Autodesk Fusion 360 part; units mm, degrees
(part 23 of 25)
sketch "Bottom Component Outlines" plane through (0, 0, 0) normal (0, 0, 1) x (1, 0, 0)
  arc A0 (46.3191, 48.2959) -> (46.3909, 48.2241) centre (46.355, 48.26) ccw
  line L0 (59.055, 7.62) -> (57.785, 7.62)
  arc A1 (67.9809, 7.5841) -> (67.9091, 7.6559) centre (67.945, 7.62) ccw
  arc A2 (67.2741, 7.0209) -> (67.3459, 6.9491) centre (67.31, 6.985) ccw
  arc A3 (52.705, 7.6708) -> (52.705, 7.5692) centre (52.705, 7.62) ccw
  arc A4 (53.9391, 5.1159) -> (54.0109, 5.0441) centre (53.975, 5.08) ccw
  arc A5 (51.3991, 5.1159) -> (51.4709, 5.0441) centre (51.435, 5.08) ccw
  arc A6 (49.4941, 7.0209) -> (49.5659, 6.9491) centre (49.53, 6.985) ccw
  arc A7 (69.215, 7.5692) -> (69.215, 7.6708) centre (69.215, 7.62) ccw
  arc A8 (49.5659, 5.7509) -> (49.4941, 5.6791) centre (49.53, 5.715) ccw
  arc A9 (52.705, 5.1308) -> (52.705, 5.0292) centre (52.705, 5.08) ccw
  arc A10 (67.9091, 5.0441) -> (67.9809, 5.1159) centre (67.945, 5.08) ccw
  arc A11 (54.5741, 6.9491) -> (54.6459, 7.0209) centre (54.61, 6.985) ccw
  line L1 (52.07, 6.985) -> (51.435, 7.62)
  line L2 (54.61, 6.985) -> (53.975, 7.62)
  line L3 (52.07, 5.715) -> (52.705, 5.08)
  line L4 (51.435, 5.08) -> (52.07, 5.715)
  arc A12 (52.7409, 7.5841) -> (52.6691, 7.6559) centre (52.705, 7.62) ccw
  arc A13 (50.1291, 5.0441) -> (50.2009, 5.1159) centre (50.165, 5.08) ccw
  arc A14 (54.6459, 5.6791) -> (54.5741, 5.7509) centre (54.61, 5.715) ccw
  arc A15 (69.7992, 5.715) -> (69.9008, 5.715) centre (69.85, 5.715) ccw
  arc A16 (51.4709, 7.6559) -> (51.3991, 7.5841) centre (51.435, 7.62) ccw
  arc A17 (46.3909, 50.8359) -> (46.3191, 50.7641) centre (46.355, 50.8) ccw
  line L5 (69.85, 6.985) -> (69.215, 7.62)
  arc A18 (52.1059, 5.7509) -> (52.0341, 5.6791) centre (52.07, 5.715) ccw
  line L6 (69.85, 5.715) -> (69.85, 6.985)
  arc A19 (69.1791, 5.1159) -> (69.2509, 5.0441) centre (69.215, 5.08) ccw
  arc A20 (54.0109, 7.6559) -> (53.9391, 7.5841) centre (53.975, 7.62) ccw
  line L7 (52.705, 5.08) -> (53.975, 5.08)
  arc A21 (52.0341, 7.0209) -> (52.1059, 6.9491) centre (52.07, 6.985) ccw
  arc A22 (69.2509, 7.6559) -> (69.1791, 7.5841) centre (69.215, 7.62) ccw
  line L8 (45.085, 48.26) -> (46.355, 48.26)
  arc A23 (52.705, 50.8508) -> (52.705, 50.7492) centre (52.705, 50.8) ccw
  arc A24 (69.9008, 6.985) -> (69.7992, 6.985) centre (69.85, 6.985) ccw
  line L9 (67.31, 6.985) -> (67.945, 7.62)
  arc A25 (53.975, 7.5692) -> (53.975, 7.6708) centre (53.975, 7.62) ccw
  line L10 (52.705, 7.62) -> (52.07, 6.985)
  arc A26 (52.1059, 5.6791) -> (52.0341, 5.7509) centre (52.07, 5.715) ccw
  arc A27 (52.6691, 5.0441) -> (52.7409, 5.1159) centre (52.705, 5.08) ccw
  line L11 (53.975, 7.62) -> (52.705, 7.62)
  arc A28 (51.435, 7.5692) -> (51.435, 7.6708) centre (51.435, 7.62) ccw
  arc A29 (67.945, 5.1308) -> (67.945, 5.0292) centre (67.945, 5.08) ccw
  line L12 (69.215, 5.08) -> (69.85, 5.715)
  arc A30 (50.165, 5.1308) -> (50.165, 5.0292) centre (50.165, 5.08) ccw
  arc A31 (57.785, 7.6708) -> (57.785, 7.5692) centre (57.785, 7.62) ccw
  arc A32 (47.0259, 48.8591) -> (46.9541, 48.9309) centre (46.99, 48.895) ccw
  arc A33 (59.055, 7.5692) -> (59.055, 7.6708) centre (59.055, 7.62) ccw
  arc A34 (69.215, 5.0292) -> (69.215, 5.1308) centre (69.215, 5.08) ccw
  arc A35 (51.435, 5.0292) -> (51.435, 5.1308) centre (51.435, 5.08) ccw
  line L13 (53.975, 5.08) -> (54.61, 5.715)
  line L14 (51.435, 7.62) -> (50.165, 7.62)
  line L15 (50.165, 5.08) -> (49.53, 5.715)
  line L16 (69.215, 7.62) -> (67.945, 7.62)
  arc A36 (67.945, 7.6708) -> (67.945, 7.5692) centre (67.945, 7.62) ccw
  line L17 (67.945, 5.08) -> (67.31, 5.715)
  arc A37 (50.2009, 7.5841) -> (50.1291, 7.6559) centre (50.165, 7.62) ccw
  arc A38 (50.165, 7.6708) -> (50.165, 7.5692) centre (50.165, 7.62) ccw
  line L18 (52.07, 48.895) -> (52.705, 48.26)
  arc A39 (52.0341, 6.9491) -> (52.1059, 7.0209) centre (52.07, 6.985) ccw
  line L19 (67.945, 5.08) -> (69.215, 5.08)
  line L20 (50.165, 5.08) -> (51.435, 5.08)
  line L21 (49.53, 6.985) -> (50.165, 7.62)
  arc A40 (67.3459, 5.7509) -> (67.2741, 5.6791) centre (67.31, 5.715) ccw
  arc A41 (69.8859, 5.6791) -> (69.8141, 5.7509) centre (69.85, 5.715) ccw
  arc A42 (52.0341, 50.2009) -> (52.1059, 50.1291) centre (52.07, 50.165) ccw
  arc A43 (46.9541, 50.2009) -> (47.0259, 50.1291) centre (46.99, 50.165) ccw
  line L22 (53.975, 50.8) -> (52.705, 50.8)
  arc A44 (46.355, 48.2092) -> (46.355, 48.3108) centre (46.355, 48.26) ccw
  arc A45 (45.0491, 48.2241) -> (45.1209, 48.2959) centre (45.085, 48.26) ccw
  arc A46 (48.895, 50.7492) -> (48.895, 50.8508) centre (48.895, 50.8) ccw
  arc A47 (45.085, 48.3108) -> (45.085, 48.2092) centre (45.085, 48.26) ccw
  line L23 (48.895, 50.8) -> (47.625, 50.8)
  line L24 (46.355, 50.8) -> (45.085, 50.8)
  line L25 (47.625, 50.8) -> (46.99, 50.165)
  arc A48 (49.4941, 50.1291) -> (49.5659, 50.2009) centre (49.53, 50.165) ccw
  line L26 (44.45, 48.895) -> (45.085, 48.26)
  arc A49 (49.5659, 48.8591) -> (49.4941, 48.9309) centre (49.53, 48.895) ccw
  arc A50 (46.9541, 50.1291) -> (47.0259, 50.2009) centre (46.99, 50.165) ccw
  arc A51 (44.4859, 48.9309) -> (44.4141, 48.8591) centre (44.45, 48.895) ccw
  arc A52 (45.1209, 50.7641) -> (45.0491, 50.8359) centre (45.085, 50.8) ccw
  arc A53 (50.2009, 50.7641) -> (50.1291, 50.8359) centre (50.165, 50.8) ccw
  arc A54 (44.4141, 50.2009) -> (44.4859, 50.1291) centre (44.45, 50.165) ccw
  line L27 (49.53, 50.165) -> (48.895, 50.8)
  line L28 (47.625, 48.26) -> (48.895, 48.26)
  line L29 (55.245, 48.26) -> (56.515, 48.26)
  arc A55 (47.0259, 48.9309) -> (46.9541, 48.8591) centre (46.99, 48.895) ccw
  line L30 (52.07, 50.165) -> (51.435, 50.8)
  line L31 (45.085, 50.8) -> (44.45, 50.165)
  arc A56 (52.7409, 50.7641) -> (52.6691, 50.8359) centre (52.705, 50.8) ccw
  arc A57 (47.6609, 50.7641) -> (47.5891, 50.8359) centre (47.625, 50.8) ccw
  arc A58 (46.355, 50.7492) -> (46.355, 50.8508) centre (46.355, 50.8) ccw
  line L32 (49.53, 48.895) -> (50.165, 48.26)
  arc A59 (55.2091, 48.2241) -> (55.2809, 48.2959) centre (55.245, 48.26) ccw
  arc A60 (47.5891, 48.2241) -> (47.6609, 48.2959) centre (47.625, 48.26) ccw
  line L33 (46.99, 48.895) -> (46.355, 48.26)
  line L34 (56.515, 50.8) -> (55.245, 50.8)
  arc A61 (53.975, 48.2092) -> (53.975, 48.3108) centre (53.975, 48.26) ccw
  arc A62 (48.8591, 48.2959) -> (48.9309, 48.2241) centre (48.895, 48.26) ccw
  arc A63 (48.895, 48.2092) -> (48.895, 48.3108) centre (48.895, 48.26) ccw
  line L35 (52.705, 50.8) -> (52.07, 50.165)
  arc A64 (47.625, 50.8508) -> (47.625, 50.7492) centre (47.625, 50.8) ccw
  arc A65 (48.9309, 50.8359) -> (48.8591, 50.7641) centre (48.895, 50.8) ccw
  arc A66 (53.975, 50.7492) -> (53.975, 50.8508) centre (53.975, 50.8) ccw
  arc A67 (45.085, 50.8508) -> (45.085, 50.7492) centre (45.085, 50.8) ccw
  arc A68 (47.625, 48.3108) -> (47.625, 48.2092) centre (47.625, 48.26) ccw
  line L36 (46.99, 48.895) -> (47.625, 48.26)
  line L37 (48.895, 48.26) -> (49.53, 48.895)
  line L38 (46.355, 50.8) -> (46.99, 50.165)
  arc A69 (59.055, 50.7492) -> (59.055, 50.8508) centre (59.055, 50.8) ccw
  arc A70 (51.435, 50.7492) -> (51.435, 50.8508) centre (51.435, 50.8) ccw
  arc A71 (50.165, 50.8508) -> (50.165, 50.7492) centre (50.165, 50.8) ccw
  arc A72 (56.515, 50.7492) -> (56.515, 50.8508) centre (56.515, 50.8) ccw
  line L39 (59.055, 50.8) -> (57.785, 50.8)
  line L40 (50.165, 50.8) -> (49.53, 50.165)
  arc A73 (59.6541, 50.1291) -> (59.7259, 50.2009) centre (59.69, 50.165) ccw
  arc A74 (61.595, 50.7492) -> (61.595, 50.8508) centre (61.595, 50.8) ccw
  arc A75 (52.1059, 48.9309) -> (52.0341, 48.8591) centre (52.07, 48.895) ccw
  line L41 (54.61, 48.895) -> (55.245, 48.26)
  arc A76 (54.6459, 48.8591) -> (54.5741, 48.9309) centre (54.61, 48.895) ccw
  arc A77 (55.245, 50.8508) -> (55.245, 50.7492) centre (55.245, 50.8) ccw
  arc A78 (60.2891, 48.2241) -> (60.3609, 48.2959) centre (60.325, 48.26) ccw
  arc A79 (52.6691, 48.2241) -> (52.7409, 48.2959) centre (52.705, 48.26) ccw
  arc A80 (60.3609, 50.7641) -> (60.2891, 50.8359) centre (60.325, 50.8) ccw
  arc A81 (52.0341, 50.1291) -> (52.1059, 50.2009) centre (52.07, 50.165) ccw
  arc A82 (51.4709, 50.8359) -> (51.3991, 50.7641) centre (51.435, 50.8) ccw
  line L42 (61.595, 50.8) -> (60.325, 50.8)
  line L43 (51.435, 50.8) -> (50.165, 50.8)
  arc A83 (57.1141, 50.1291) -> (57.1859, 50.2009) centre (57.15, 50.165) ccw
  line L44 (57.15, 50.165) -> (56.515, 50.8)
  arc A84 (50.165, 48.3108) -> (50.165, 48.2092) centre (50.165, 48.26) ccw
  arc A85 (55.2809, 50.7641) -> (55.2091, 50.8359) centre (55.245, 50.8) ccw
  line L45 (51.435, 48.26) -> (52.07, 48.895)
  arc A86 (57.1141, 50.2009) -> (57.1859, 50.1291) centre (57.15, 50.165) ccw
  arc A87 (51.435, 48.2092) -> (51.435, 48.3108) centre (51.435, 48.26) ccw
  arc A88 (55.245, 48.3108) -> (55.245, 48.2092) centre (55.245, 48.26) ccw
  arc A89 (52.705, 48.3108) -> (52.705, 48.2092) centre (52.705, 48.26) ccw
  arc A90 (60.325, 50.8508) -> (60.325, 50.7492) centre (60.325, 50.8) ccw
  line L46 (59.69, 48.895) -> (60.325, 48.26)
  arc A91 (49.5659, 48.9309) -> (49.4941, 48.8591) centre (49.53, 48.895) ccw
  line L47 (54.61, 48.895) -> (53.975, 48.26)
  line L48 (50.165, 48.26) -> (51.435, 48.26)
  line L49 (57.785, 50.8) -> (57.15, 50.165)
  arc A92 (56.5509, 50.8359) -> (56.4791, 50.7641) centre (56.515, 50.8) ccw
  arc A93 (54.5741, 50.1291) -> (54.6459, 50.2009) centre (54.61, 50.165) ccw
  arc A94 (49.4941, 50.2009) -> (49.5659, 50.1291) centre (49.53, 50.165) ccw
  arc A95 (53.9391, 48.2959) -> (54.0109, 48.2241) centre (53.975, 48.26) ccw
  arc A96 (52.1059, 48.8591) -> (52.0341, 48.9309) centre (52.07, 48.895) ccw
  line L50 (52.705, 48.26) -> (53.975, 48.26)
  arc A97 (54.6459, 48.9309) -> (54.5741, 48.8591) centre (54.61, 48.895) ccw
  arc A98 (54.5741, 50.2009) -> (54.6459, 50.1291) centre (54.61, 50.165) ccw
  arc A99 (57.785, 50.8508) -> (57.785, 50.7492) centre (57.785, 50.8) ccw
  arc A100 (57.1859, 48.8591) -> (57.1141, 48.9309) centre (57.15, 48.895) ccw
  arc A101 (59.0191, 48.2959) -> (59.0909, 48.2241) centre (59.055, 48.26) ccw
  arc A102 (51.3991, 48.2959) -> (51.4709, 48.2241) centre (51.435, 48.26) ccw
  line L51 (57.785, 48.26) -> (59.055, 48.26)
  line L52 (60.325, 50.8) -> (59.69, 50.165)
  arc A103 (54.0109, 50.8359) -> (53.9391, 50.7641) centre (53.975, 50.8) ccw
  line L53 (56.515, 48.26) -> (57.15, 48.895)
  line L54 (59.69, 50.165) -> (59.055, 50.8)
  arc A104 (59.0909, 50.8359) -> (59.0191, 50.7641) centre (59.055, 50.8) ccw
  line L55 (55.245, 50.8) -> (54.61, 50.165)
  arc A105 (28.575, 50.7492) -> (28.575, 50.8508) centre (28.575, 50.8) ccw
  arc A106 (26.7059, 48.9309) -> (26.6341, 48.8591) centre (26.67, 48.895) ccw
  arc A107 (29.2459, 48.9309) -> (29.1741, 48.8591) centre (29.21, 48.895) ccw
  arc A108 (26.6341, 50.2009) -> (26.7059, 50.1291) centre (26.67, 50.165) ccw
  arc A109 (31.1509, 50.8359) -> (31.0791, 50.7641) centre (31.115, 50.8) ccw
  line L56 (34.925, 50.8) -> (34.29, 50.165)
  arc A110 (56.4791, 48.2959) -> (56.5509, 48.2241) centre (56.515, 48.26) ccw
  line L57 (28.575, 50.8) -> (29.21, 50.165)
  arc A111 (56.515, 48.2092) -> (56.515, 48.3108) centre (56.515, 48.26) ccw
  arc A112 (57.785, 48.3108) -> (57.785, 48.2092) centre (57.785, 48.26) ccw
  arc A113 (62.2659, 48.8591) -> (62.1941, 48.9309) centre (62.23, 48.895) ccw
  line L58 (29.21, 48.895) -> (28.575, 48.26)
  arc A114 (29.1741, 50.2009) -> (29.2459, 50.1291) centre (29.21, 50.165) ccw
  line L59 (59.055, 48.26) -> (59.69, 48.895)
  line L60 (29.845, 48.26) -> (31.115, 48.26)
  arc A115 (50.1291, 48.2241) -> (50.2009, 48.2959) centre (50.165, 48.26) ccw
  arc A116 (62.1941, 50.1291) -> (62.2659, 50.2009) centre (62.23, 50.165) ccw
  arc A117 (62.1792, 48.895) -> (62.2808, 48.895) centre (62.23, 48.895) ccw
  arc A118 (34.9609, 50.7641) -> (34.8891, 50.8359) centre (34.925, 50.8) ccw
  arc A119 (31.115, 48.2092) -> (31.115, 48.3108) centre (31.115, 48.26) ccw
  line L61 (29.845, 50.8) -> (29.21, 50.165)
  line L62 (31.75, 50.165) -> (31.115, 50.8)
  line L63 (27.305, 50.8) -> (26.67, 50.165)
  arc A120 (59.6541, 50.2009) -> (59.7259, 50.1291) centre (59.69, 50.165) ccw
  arc A121 (27.3409, 50.7641) -> (27.2691, 50.8359) centre (27.305, 50.8) ccw
  arc A122 (57.7491, 48.2241) -> (57.8209, 48.2959) centre (57.785, 48.26) ccw
  arc A123 (34.2541, 50.2009) -> (34.3259, 50.1291) centre (34.29, 50.165) ccw
  arc A124 (61.595, 48.2092) -> (61.595, 48.3108) centre (61.595, 48.26) ccw
  arc A125 (31.115, 50.7492) -> (31.115, 50.8508) centre (31.115, 50.8) ccw
  line L64 (53.975, 50.8) -> (54.61, 50.165)
  arc A126 (62.2808, 50.165) -> (62.1792, 50.165) centre (62.23, 50.165) ccw
  arc A127 (59.7259, 48.9309) -> (59.6541, 48.8591) centre (59.69, 48.895) ccw
  arc A128 (34.925, 50.8508) -> (34.925, 50.7492) centre (34.925, 50.8) ccw
  line L65 (62.23, 50.165) -> (62.23, 48.895)
  line L66 (62.23, 48.895) -> (61.595, 48.26)
  arc A129 (59.7259, 48.8591) -> (59.6541, 48.9309) centre (59.69, 48.895) ccw
  arc A130 (36.8659, 48.8591) -> (36.7941, 48.9309) centre (36.83, 48.895) ccw
  arc A131 (37.465, 48.3108) -> (37.465, 48.2092) centre (37.465, 48.26) ccw
  arc A132 (36.8659, 48.9309) -> (36.7941, 48.8591) centre (36.83, 48.895) ccw
  arc A133 (39.4059, 48.8591) -> (39.3341, 48.9309) centre (39.37, 48.895) ccw
  line L67 (57.15, 48.895) -> (57.785, 48.26)
  arc A134 (60.325, 48.3108) -> (60.325, 48.2092) centre (60.325, 48.26) ccw
  arc A135 (29.8809, 50.7641) -> (29.8091, 50.8359) centre (29.845, 50.8) ccw
  arc A136 (29.2459, 48.8591) -> (29.1741, 48.9309) centre (29.21, 48.895) ccw
  line L68 (60.325, 48.26) -> (61.595, 48.26)
  line L69 (29.21, 48.895) -> (29.845, 48.26)
  line L70 (31.115, 48.26) -> (31.75, 48.895)
  arc A137 (29.845, 50.8508) -> (29.845, 50.7492) centre (29.845, 50.8) ccw
  arc A138 (61.5591, 48.2959) -> (61.6309, 48.2241) centre (61.595, 48.26) ccw
  arc A139 (34.3259, 48.8591) -> (34.2541, 48.9309) centre (34.29, 48.895) ccw
  line L71 (34.29, 50.165) -> (33.655, 50.8)
  arc A140 (43.815, 50.7492) -> (43.815, 50.8508) centre (43.815, 50.8) ccw
  arc A141 (57.8209, 50.7641) -> (57.7491, 50.8359) centre (57.785, 50.8) ccw
  line L72 (32.385, 50.8) -> (31.75, 50.165)
  arc A142 (61.6309, 50.8359) -> (61.5591, 50.7641) centre (61.595, 50.8) ccw
  line L73 (27.305, 48.26) -> (28.575, 48.26)
  arc A143 (27.305, 50.8508) -> (27.305, 50.7492) centre (27.305, 50.8) ccw
  line L74 (36.195, 50.8) -> (36.83, 50.165)
  line L75 (31.115, 50.8) -> (29.845, 50.8)
  arc A144 (28.5391, 48.2959) -> (28.6109, 48.2241) centre (28.575, 48.26) ccw
  arc A145 (31.7141, 50.1291) -> (31.7859, 50.2009) centre (31.75, 50.165) ccw
  arc A146 (29.8091, 48.2241) -> (29.8809, 48.2959) centre (29.845, 48.26) ccw
  line L76 (26.67, 48.895) -> (27.305, 48.26)
  arc A147 (57.1859, 48.9309) -> (57.1141, 48.8591) centre (57.15, 48.895) ccw
  arc A148 (31.7859, 48.8591) -> (31.7141, 48.9309) centre (31.75, 48.895) ccw
  arc A149 (34.2541, 50.1291) -> (34.3259, 50.2009) centre (34.29, 50.165) ccw
  line L77 (28.575, 50.8) -> (27.305, 50.8)
  line L78 (36.195, 50.8) -> (34.925, 50.8)
  arc A150 (29.1741, 50.1291) -> (29.2459, 50.2009) centre (29.21, 50.165) ccw
  arc A151 (31.0791, 48.2959) -> (31.1509, 48.2241) centre (31.115, 48.26) ccw
  arc A152 (27.2691, 48.2241) -> (27.3409, 48.2959) centre (27.305, 48.26) ccw
  arc A153 (36.195, 50.7492) -> (36.195, 50.8508) centre (36.195, 50.8) ccw
  line L79 (36.83, 48.895) -> (37.465, 48.26)
  arc A154 (28.6109, 50.8359) -> (28.5391, 50.7641) centre (28.575, 50.8) ccw
  line L80 (33.655, 50.8) -> (32.385, 50.8)
  arc A155 (41.9459, 48.9309) -> (41.8741, 48.8591) centre (41.91, 48.895) ccw
  arc A156 (29.845, 48.3108) -> (29.845, 48.2092) centre (29.845, 48.26) ccw
  arc A157 (59.055, 48.2092) -> (59.055, 48.3108) centre (59.055, 48.26) ccw
  line L81 (61.595, 50.8) -> (62.23, 50.165)
  arc A158 (28.575, 48.2092) -> (28.575, 48.3108) centre (28.575, 48.26) ccw
  arc A159 (27.305, 48.3108) -> (27.305, 48.2092) centre (27.305, 48.26) ccw
  arc A160 (32.385, 48.3108) -> (32.385, 48.2092) centre (32.385, 48.26) ccw
  line L82 (34.29, 48.895) -> (34.925, 48.26)
  arc A161 (42.5809, 50.7641) -> (42.5091, 50.8359) centre (42.545, 50.8) ccw
  line L83 (31.75, 48.895) -> (32.385, 48.26)
  arc A162 (42.545, 50.8508) -> (42.545, 50.7492) centre (42.545, 50.8) ccw
  line L84 (32.385, 48.26) -> (33.655, 48.26)
  line L85 (33.655, 48.26) -> (34.29, 48.895)
  arc A163 (39.3341, 50.1291) -> (39.4059, 50.2009) centre (39.37, 50.165) ccw
  line L86 (41.91, 48.895) -> (42.545, 48.26)
  arc A164 (33.655, 50.7492) -> (33.655, 50.8508) centre (33.655, 50.8) ccw
  arc A165 (42.5091, 48.2241) -> (42.5809, 48.2959) centre (42.545, 48.26) ccw
  arc A166 (41.3109, 50.8359) -> (41.2391, 50.7641) centre (41.275, 50.8) ccw
  line L87 (43.815, 50.8) -> (42.545, 50.8)
  arc A167 (36.2309, 50.8359) -> (36.1591, 50.7641) centre (36.195, 50.8) ccw
  arc A168 (34.8891, 48.2241) -> (34.9609, 48.2959) centre (34.925, 48.26) ccw
  arc A169 (38.7709, 50.8359) -> (38.6991, 50.7641) centre (38.735, 50.8) ccw
  line L88 (38.735, 48.26) -> (39.37, 48.895)
  arc A170 (36.1591, 48.2959) -> (36.2309, 48.2241) centre (36.195, 48.26) ccw
  line L89 (41.91, 50.165) -> (41.275, 50.8)
  arc A171 (32.3491, 48.2241) -> (32.4209, 48.2959) centre (32.385, 48.26) ccw
  arc A172 (33.6909, 50.8359) -> (33.6191, 50.7641) centre (33.655, 50.8) ccw
  line L90 (40.005, 50.8) -> (39.37, 50.165)
  line L91 (36.83, 48.895) -> (36.195, 48.26)
  line L92 (42.545, 50.8) -> (41.91, 50.165)
  arc A173 (33.655, 48.2092) -> (33.655, 48.3108) centre (33.655, 48.26) ccw
  arc A174 (33.6191, 48.2959) -> (33.6909, 48.2241) centre (33.655, 48.26) ccw
  arc A175 (32.4209, 50.7641) -> (32.3491, 50.8359) centre (32.385, 50.8) ccw
  line L93 (37.465, 50.8) -> (36.83, 50.165)
  arc A176 (31.7859, 48.9309) -> (31.7141, 48.8591) centre (31.75, 48.895) ccw
  line L94 (34.925, 48.26) -> (36.195, 48.26)
  arc A177 (36.195, 48.2092) -> (36.195, 48.3108) centre (36.195, 48.26) ccw
  arc A178 (36.7941, 50.1291) -> (36.8659, 50.2009) centre (36.83, 50.165) ccw
  line L95 (38.735, 50.8) -> (37.465, 50.8)
  arc A179 (34.925, 48.3108) -> (34.925, 48.2092) centre (34.925, 48.26) ccw
  arc A180 (37.5009, 50.7641) -> (37.4291, 50.8359) centre (37.465, 50.8) ccw
  arc A181 (31.7141, 50.2009) -> (31.7859, 50.1291) centre (31.75, 50.165) ccw
  arc A182 (38.735, 48.2092) -> (38.735, 48.3108) centre (38.735, 48.26) ccw
  arc A183 (40.005, 50.8508) -> (40.005, 50.7492) centre (40.005, 50.8) ccw
  arc A184 (37.465, 50.8508) -> (37.465, 50.7492) centre (37.465, 50.8) ccw
  arc A185 (41.8741, 50.2009) -> (41.9459, 50.1291) centre (41.91, 50.165) ccw
  line L96 (37.465, 48.26) -> (38.735, 48.26)
  arc A186 (38.6991, 48.2959) -> (38.7709, 48.2241) centre (38.735, 48.26) ccw
  arc A187 (34.3259, 48.9309) -> (34.2541, 48.8591) centre (34.29, 48.895) ccw
  arc A188 (41.275, 50.7492) -> (41.275, 50.8508) centre (41.275, 50.8) ccw
  arc A189 (43.815, 48.2092) -> (43.815, 48.3108) centre (43.815, 48.26) ccw
  line L97 (39.37, 50.165) -> (38.735, 50.8)
  arc A190 (41.8741, 50.1291) -> (41.9459, 50.2009) centre (41.91, 50.165) ccw
  line L98 (41.275, 50.8) -> (40.005, 50.8)
  arc A191 (36.7941, 50.2009) -> (36.8659, 50.1291) centre (36.83, 50.165) ccw
  arc A192 (32.385, 50.8508) -> (32.385, 50.7492) centre (32.385, 50.8) ccw
  arc A193 (38.735, 50.7492) -> (38.735, 50.8508) centre (38.735, 50.8) ccw
  line L99 (44.45, 48.895) -> (43.815, 48.26)
  arc A194 (37.4291, 48.2241) -> (37.5009, 48.2959) centre (37.465, 48.26) ccw
  line L100 (42.545, 48.26) -> (43.815, 48.26)
  line L101 (24.765, 48.26) -> (26.035, 48.26)
  arc A195 (44.4141, 50.1291) -> (44.4859, 50.2009) centre (44.45, 50.165) ccw
  arc A196 (43.7791, 48.2959) -> (43.8509, 48.2241) centre (43.815, 48.26) ccw
  arc A197 (26.035, 48.2092) -> (26.035, 48.3108) centre (26.035, 48.26) ccw
  line L102 (40.005, 48.26) -> (41.275, 48.26)
  line L103 (41.275, 48.26) -> (41.91, 48.895)
  arc A198 (24.765, 48.3108) -> (24.765, 48.2092) centre (24.765, 48.26) ccw
  arc A199 (24.0941, 50.2009) -> (24.1659, 50.1291) centre (24.13, 50.165) ccw
  arc A200 (24.1808, 50.165) -> (24.0792, 50.165) centre (24.13, 50.165) ccw
  arc A201 (25.9991, 48.2959) -> (26.0709, 48.2241) centre (26.035, 48.26) ccw
  line L104 (24.13, 48.895) -> (24.765, 48.26)
  arc A202 (24.8009, 50.7641) -> (24.7291, 50.8359) centre (24.765, 50.8) ccw
  line L105 (39.37, 48.895) -> (40.005, 48.26)
  line L106 (26.035, 50.8) -> (26.67, 50.165)
  arc A203 (39.4059, 48.9309) -> (39.3341, 48.8591) centre (39.37, 48.895) ccw
  line L107 (24.765, 50.8) -> (24.13, 50.165)
  arc A204 (26.7059, 48.8591) -> (26.6341, 48.9309) centre (26.67, 48.895) ccw
  line L108 (26.035, 50.8) -> (24.765, 50.8)
  arc A205 (40.005, 48.3108) -> (40.005, 48.2092) centre (40.005, 48.26) ccw
  arc A206 (41.275, 48.2092) -> (41.275, 48.3108) centre (41.275, 48.26) ccw
  arc A207 (24.765, 50.8508) -> (24.765, 50.7492) centre (24.765, 50.8) ccw
  line L109 (43.815, 50.8) -> (44.45, 50.165)
  arc A208 (24.0792, 48.895) -> (24.1808, 48.895) centre (24.13, 48.895) ccw
  arc A209 (24.1659, 48.9309) -> (24.0941, 48.8591) centre (24.13, 48.895) ccw
  arc A210 (40.0409, 50.7641) -> (39.9691, 50.8359) centre (40.005, 50.8) ccw
  arc A211 (24.7291, 48.2241) -> (24.8009, 48.2959) centre (24.765, 48.26) ccw
  arc A212 (26.035, 50.7492) -> (26.035, 50.8508) centre (26.035, 50.8) ccw
  arc A213 (39.9691, 48.2241) -> (40.0409, 48.2959) centre (40.005, 48.26) ccw
  arc A214 (43.8509, 50.8359) -> (43.7791, 50.7641) centre (43.815, 50.8) ccw
  arc A215 (26.0709, 50.8359) -> (25.9991, 50.7641) centre (26.035, 50.8) ccw
  arc A216 (42.545, 48.3108) -> (42.545, 48.2092) centre (42.545, 48.26) ccw
  arc A217 (41.9459, 48.8591) -> (41.8741, 48.9309) centre (41.91, 48.895) ccw
  arc A218 (26.6341, 50.1291) -> (26.7059, 50.2009) centre (26.67, 50.165) ccw
  arc A219 (44.4859, 48.8591) -> (44.4141, 48.9309) centre (44.45, 48.895) ccw
  line L110 (24.13, 50.165) -> (24.13, 48.895)
  arc A220 (39.3341, 50.2009) -> (39.4059, 50.1291) centre (39.37, 50.165) ccw
  arc A221 (41.2391, 48.2959) -> (41.3109, 48.2241) centre (41.275, 48.26) ccw
  line L111 (26.67, 48.895) -> (26.035, 48.26)
  arc A222 (49.5659, 5.6791) -> (49.4941, 5.7509) centre (49.53, 5.715) ccw
  arc A223 (46.3191, 5.1159) -> (46.3909, 5.0441) centre (46.355, 5.08) ccw
  line L112 (48.895, 5.08) -> (49.53, 5.715)
  arc A224 (46.3909, 7.6559) -> (46.3191, 7.5841) centre (46.355, 7.62) ccw
  arc A225 (47.0259, 5.6791) -> (46.9541, 5.7509) centre (46.99, 5.715) ccw
  arc A226 (37.5009, 7.5841) -> (37.4291, 7.6559) centre (37.465, 7.62) ccw
  line L113 (41.91, 5.715) -> (42.545, 5.08)
  line L114 (40.005, 5.08) -> (39.37, 5.715)
  arc A227 (39.9691, 5.0441) -> (40.0409, 5.1159) centre (40.005, 5.08) ccw
  line L115 (46.99, 6.985) -> (46.355, 7.62)
  line L116 (46.355, 7.62) -> (45.085, 7.62)
  arc A228 (47.625, 5.1308) -> (47.625, 5.0292) centre (47.625, 5.08) ccw
  arc A229 (46.355, 5.0292) -> (46.355, 5.1308) centre (46.355, 5.08) ccw
  arc A230 (44.4859, 5.7509) -> (44.4141, 5.6791) centre (44.45, 5.715) ccw
  line L117 (47.625, 5.08) -> (48.895, 5.08)
  arc A231 (49.4941, 6.9491) -> (49.5659, 7.0209) centre (49.53, 6.985) ccw
  arc A232 (46.9541, 6.9491) -> (47.0259, 7.0209) centre (46.99, 6.985) ccw
  arc A233 (48.8591, 5.1159) -> (48.9309, 5.0441) centre (48.895, 5.08) ccw
  arc A234 (46.355, 7.5692) -> (46.355, 7.6708) centre (46.355, 7.62) ccw
  line L118 (46.355, 5.08) -> (46.99, 5.715)
  line L119 (44.45, 5.715) -> (45.085, 5.08)
  arc A235 (45.0491, 5.0441) -> (45.1209, 5.1159) centre (45.085, 5.08) ccw
  line L120 (46.99, 6.985) -> (47.625, 7.62)
  arc A236 (48.895, 5.0292) -> (48.895, 5.1308) centre (48.895, 5.08) ccw
  line L121 (37.465, 7.62) -> (36.83, 6.985)
  arc A237 (45.085, 7.6708) -> (45.085, 7.5692) centre (45.085, 7.62) ccw
  arc A238 (48.9309, 7.6559) -> (48.8591, 7.5841) centre (48.895, 7.62) ccw
  arc A239 (44.4859, 5.6791) -> (44.4141, 5.7509) centre (44.45, 5.715) ccw
  arc A240 (47.6609, 7.5841) -> (47.5891, 7.6559) centre (47.625, 7.62) ccw
  line L122 (45.085, 5.08) -> (46.355, 5.08)
  arc A241 (42.545, 5.1308) -> (42.545, 5.0292) centre (42.545, 5.08) ccw
  arc A242 (40.005, 5.1308) -> (40.005, 5.0292) centre (40.005, 5.08) ccw
  arc A243 (38.735, 5.0292) -> (38.735, 5.1308) centre (38.735, 5.08) ccw
  line L123 (49.53, 6.985) -> (48.895, 7.62)
  arc A244 (45.085, 5.1308) -> (45.085, 5.0292) centre (45.085, 5.08) ccw
  arc A245 (43.815, 7.5692) -> (43.815, 7.6708) centre (43.815, 7.62) ccw
  arc A246 (47.0259, 5.7509) -> (46.9541, 5.6791) centre (46.99, 5.715) ccw
  arc A247 (39.4059, 5.7509) -> (39.3341, 5.6791) centre (39.37, 5.715) ccw
  line L124 (42.545, 7.62) -> (41.91, 6.985)
  arc A248 (41.3109, 7.6559) -> (41.2391, 7.5841) centre (41.275, 7.62) ccw
  line L125 (41.275, 7.62) -> (40.005, 7.62)
  line L126 (48.895, 7.62) -> (47.625, 7.62)
  arc A249 (38.735, 7.5692) -> (38.735, 7.6708) centre (38.735, 7.62) ccw
  arc A250 (38.7709, 7.6559) -> (38.6991, 7.5841) centre (38.735, 7.62) ccw
  arc A251 (41.275, 5.0292) -> (41.275, 5.1308) centre (41.275, 5.08) ccw
  line L127 (37.465, 5.08) -> (38.735, 5.08)
  arc A252 (36.8659, 5.7509) -> (36.7941, 5.6791) centre (36.83, 5.715) ccw
  arc A253 (39.3341, 7.0209) -> (39.4059, 6.9491) centre (39.37, 6.985) ccw
  arc A254 (41.9459, 5.7509) -> (41.8741, 5.6791) centre (41.91, 5.715) ccw
  line L128 (38.735, 5.08) -> (39.37, 5.715)
  arc A255 (45.1209, 7.5841) -> (45.0491, 7.6559) centre (45.085, 7.62) ccw
  arc A256 (42.5091, 5.0441) -> (42.5809, 5.1159) centre (42.545, 5.08) ccw
  arc A257 (43.8509, 7.6559) -> (43.7791, 7.5841) centre (43.815, 7.62) ccw
  line L129 (43.815, 7.62) -> (42.545, 7.62)
  arc A258 (43.7791, 5.1159) -> (43.8509, 5.0441) centre (43.815, 5.08) ccw
  arc A259 (48.895, 7.5692) -> (48.895, 7.6708) centre (48.895, 7.62) ccw
  arc A260 (37.465, 5.1308) -> (37.465, 5.0292) centre (37.465, 5.08) ccw
  arc A261 (41.9459, 5.6791) -> (41.8741, 5.7509) centre (41.91, 5.715) ccw
  line L130 (38.735, 7.62) -> (37.465, 7.62)
  arc A262 (37.4291, 5.0441) -> (37.5009, 5.1159) centre (37.465, 5.08) ccw
  arc A263 (34.2541, 6.9491) -> (34.3259, 7.0209) centre (34.29, 6.985) ccw
  arc A264 (36.1591, 5.1159) -> (36.2309, 5.0441) centre (36.195, 5.08) ccw
  line L131 (47.625, 5.08) -> (46.99, 5.715)
  arc A265 (42.545, 7.6708) -> (42.545, 7.5692) centre (42.545, 7.62) ccw
  arc A266 (41.2391, 5.1159) -> (41.3109, 5.0441) centre (41.275, 5.08) ccw
  line L132 (42.545, 5.08) -> (43.815, 5.08)
  arc A267 (41.8741, 7.0209) -> (41.9459, 6.9491) centre (41.91, 6.985) ccw
  arc A268 (34.9609, 7.5841) -> (34.8891, 7.6559) centre (34.925, 7.62) ccw
  line L133 (31.75, 5.715) -> (31.75, 6.985)
  arc A269 (31.7859, 5.7509) -> (31.7141, 5.6791) centre (31.75, 5.715) ccw
  arc A270 (36.8659, 5.6791) -> (36.7941, 5.7509) centre (36.83, 5.715) ccw
  arc A271 (46.9541, 7.0209) -> (47.0259, 6.9491) centre (46.99, 6.985) ccw
  arc A272 (47.625, 7.6708) -> (47.625, 7.5692) centre (47.625, 7.62) ccw
  arc A273 (39.4059, 5.6791) -> (39.3341, 5.7509) centre (39.37, 5.715) ccw
  arc A274 (38.6991, 5.1159) -> (38.7709, 5.0441) centre (38.735, 5.08) ccw
  line L134 (39.37, 6.985) -> (38.735, 7.62)
  arc A275 (37.465, 7.6708) -> (37.465, 7.5692) centre (37.465, 7.62) ccw
  arc A276 (34.8891, 5.0441) -> (34.9609, 5.1159) centre (34.925, 5.08) ccw
  arc A277 (36.7941, 7.0209) -> (36.8659, 6.9491) centre (36.83, 6.985) ccw
  line L135 (41.91, 6.985) -> (41.275, 7.62)
  arc A278 (36.2309, 7.6559) -> (36.1591, 7.5841) centre (36.195, 7.62) ccw
  arc A279 (31.8008, 6.985) -> (31.6992, 6.985) centre (31.75, 6.985) ccw
  line L136 (45.085, 7.62) -> (44.45, 6.985)
  line L137 (36.83, 5.715) -> (37.465, 5.08)
  line L138 (43.815, 5.08) -> (44.45, 5.715)
  line L139 (41.275, 5.08) -> (41.91, 5.715)
  arc A280 (44.4141, 6.9491) -> (44.4859, 7.0209) centre (44.45, 6.985) ccw
  line L140 (40.005, 5.08) -> (41.275, 5.08)
  arc A281 (42.5809, 7.5841) -> (42.5091, 7.6559) centre (42.545, 7.62) ccw
  line L141 (34.925, 7.62) -> (34.29, 6.985)
  line L142 (44.45, 6.985) -> (43.815, 7.62)
  line L143 (39.37, 6.985) -> (40.005, 7.62)
  arc A282 (32.3491, 5.0441) -> (32.4209, 5.1159) centre (32.385, 5.08) ccw
  arc A283 (34.3259, 5.7509) -> (34.2541, 5.6791) centre (34.29, 5.715) ccw
  arc A284 (32.385, 5.1308) -> (32.385, 5.0292) centre (32.385, 5.08) ccw
  arc A285 (32.4209, 7.5841) -> (32.3491, 7.6559) centre (32.385, 7.62) ccw
  arc A286 (39.3341, 6.9491) -> (39.4059, 7.0209) centre (39.37, 6.985) ccw
  arc A287 (43.815, 5.0292) -> (43.815, 5.1308) centre (43.815, 5.08) ccw
  arc A288 (41.8741, 6.9491) -> (41.9459, 7.0209) centre (41.91, 6.985) ccw
  arc A289 (40.0409, 7.5841) -> (39.9691, 7.6559) centre (40.005, 7.62) ccw
  arc A290 (47.5891, 5.0441) -> (47.6609, 5.1159) centre (47.625, 5.08) ccw
  arc A291 (44.4141, 7.0209) -> (44.4859, 6.9491) centre (44.45, 6.985) ccw
  arc A292 (64.8059, 5.6791) -> (64.7341, 5.7509) centre (64.77, 5.715) ccw
  line L144 (66.675, 5.08) -> (67.31, 5.715)
  arc A293 (61.595, 5.0292) -> (61.595, 5.1308) centre (61.595, 5.08) ccw
  arc A294 (64.7341, 6.9491) -> (64.8059, 7.0209) centre (64.77, 6.985) ccw
  arc A295 (34.3259, 5.6791) -> (34.2541, 5.7509) centre (34.29, 5.715) ccw
  arc A296 (36.195, 5.0292) -> (36.195, 5.1308) centre (36.195, 5.08) ccw
  arc A297 (64.0991, 5.1159) -> (64.1709, 5.0441) centre (64.135, 5.08) ccw
  arc A298 (66.7109, 7.6559) -> (66.6391, 7.5841) centre (66.675, 7.62) ccw
  arc A299 (34.925, 5.1308) -> (34.925, 5.0292) centre (34.925, 5.08) ccw
  line L145 (64.77, 6.985) -> (64.135, 7.62)
  line L146 (36.83, 6.985) -> (36.195, 7.62)
  arc A300 (64.1709, 7.6559) -> (64.0991, 7.5841) centre (64.135, 7.62) ccw
  arc A301 (36.195, 7.5692) -> (36.195, 7.6708) centre (36.195, 7.62) ccw
  arc A302 (33.6191, 5.1159) -> (33.6909, 5.0441) centre (33.655, 5.08) ccw
  arc A303 (66.6391, 5.1159) -> (66.7109, 5.0441) centre (66.675, 5.08) ccw
  line L147 (34.925, 5.08) -> (36.195, 5.08)
  arc A304 (34.2541, 7.0209) -> (34.3259, 6.9491) centre (34.29, 6.985) ccw
  line L148 (62.865, 5.08) -> (64.135, 5.08)
  arc A305 (32.385, 7.6708) -> (32.385, 7.5692) centre (32.385, 7.62) ccw
  arc A306 (67.2741, 6.9491) -> (67.3459, 7.0209) centre (67.31, 6.985) ccw
  arc A307 (33.655, 7.5692) -> (33.655, 7.6708) centre (33.655, 7.62) ccw
  arc A308 (40.005, 7.6708) -> (40.005, 7.5692) centre (40.005, 7.62) ccw
  arc A309 (36.7941, 6.9491) -> (36.8659, 7.0209) centre (36.83, 6.985) ccw
  line L149 (62.23, 5.715) -> (62.865, 5.08)
  arc A310 (62.2659, 5.7509) -> (62.1941, 5.6791) centre (62.23, 5.715) ccw
  line L150 (55.245, 5.08) -> (56.515, 5.08)
  arc A311 (67.3459, 5.6791) -> (67.2741, 5.7509) centre (67.31, 5.715) ccw
  arc A312 (62.865, 5.1308) -> (62.865, 5.0292) centre (62.865, 5.08) ccw
  line L151 (54.61, 5.715) -> (55.245, 5.08)
  line L152 (56.515, 5.08) -> (57.15, 5.715)
  arc A313 (65.4409, 7.5841) -> (65.3691, 7.6559) centre (65.405, 7.62) ccw
  arc A314 (59.055, 5.0292) -> (59.055, 5.1308) centre (59.055, 5.08) ccw
  line L153 (34.29, 6.985) -> (33.655, 7.62)
  arc A315 (33.6909, 7.6559) -> (33.6191, 7.5841) centre (33.655, 7.62) ccw
  line L154 (31.75, 6.985) -> (32.385, 7.62)
  line L155 (59.69, 5.715) -> (60.325, 5.08)
  arc A316 (57.1859, 5.6791) -> (57.1141, 5.7509) centre (57.15, 5.715) ccw
  arc A317 (59.0191, 5.1159) -> (59.0909, 5.0441) centre (59.055, 5.08) ccw
  arc A318 (56.5509, 7.6559) -> (56.4791, 7.5841) centre (56.515, 7.62) ccw
  line L156 (32.385, 5.08) -> (33.655, 5.08)
  arc A319 (54.6459, 5.7509) -> (54.5741, 5.6791) centre (54.61, 5.715) ccw
  line L157 (36.195, 5.08) -> (36.83, 5.715)
  line L158 (33.655, 5.08) -> (34.29, 5.715)
  line L159 (32.385, 5.08) -> (31.75, 5.715)
  line L160 (57.15, 6.985) -> (56.515, 7.62)
  arc A320 (55.245, 5.1308) -> (55.245, 5.0292) centre (55.245, 5.08) ccw
  arc A321 (34.925, 7.6708) -> (34.925, 7.5692) centre (34.925, 7.62) ccw
  arc A322 (31.7141, 7.0209) -> (31.7859, 6.9491) centre (31.75, 6.985) ccw
  line L161 (64.135, 5.08) -> (64.77, 5.715)
  arc A323 (41.275, 7.5692) -> (41.275, 7.6708) centre (41.275, 7.62) ccw
  arc A324 (65.405, 5.1308) -> (65.405, 5.0292) centre (65.405, 5.08) ccw
  line L162 (67.31, 6.985) -> (66.675, 7.62)
  arc A325 (64.135, 5.0292) -> (64.135, 5.1308) centre (64.135, 5.08) ccw
  arc A326 (33.655, 5.0292) -> (33.655, 5.1308) centre (33.655, 5.08) ccw
  line L163 (59.055, 5.08) -> (59.69, 5.715)
  line L164 (65.405, 5.08) -> (66.675, 5.08)
  arc A327 (62.8291, 5.0441) -> (62.9009, 5.1159) centre (62.865, 5.08) ccw
  arc A328 (66.675, 5.0292) -> (66.675, 5.1308) centre (66.675, 5.08) ccw
  line L165 (33.655, 7.62) -> (32.385, 7.62)
  line L166 (34.29, 5.715) -> (34.925, 5.08)
  line L167 (36.195, 7.62) -> (34.925, 7.62)
  line L168 (64.135, 7.62) -> (62.865, 7.62)
  arc A329 (62.865, 7.6708) -> (62.865, 7.5692) centre (62.865, 7.62) ccw
  arc A330 (31.6992, 5.715) -> (31.8008, 5.715) centre (31.75, 5.715) ccw
  line L169 (56.515, 7.62) -> (55.245, 7.62)
  line L170 (57.785, 5.08) -> (59.055, 5.08)
  arc A331 (57.7491, 5.0441) -> (57.8209, 5.1159) centre (57.785, 5.08) ccw
  arc A332 (64.135, 7.5692) -> (64.135, 7.6708) centre (64.135, 7.62) ccw
  arc A333 (62.2659, 5.6791) -> (62.1941, 5.7509) centre (62.23, 5.715) ccw
  arc A334 (65.405, 7.6708) -> (65.405, 7.5692) centre (65.405, 7.62) ccw
  arc A335 (59.0909, 7.6559) -> (59.0191, 7.5841) centre (59.055, 7.62) ccw
  arc A336 (54.5741, 7.0209) -> (54.6459, 6.9491) centre (54.61, 6.985) ccw
  arc A337 (61.595, 7.5692) -> (61.595, 7.6708) centre (61.595, 7.62) ccw
  line L171 (60.325, 7.62) -> (59.69, 6.985)
  arc A338 (64.8059, 5.7509) -> (64.7341, 5.6791) centre (64.77, 5.715) ccw
  arc A339 (56.4791, 5.1159) -> (56.5509, 5.0441) centre (56.515, 5.08) ccw
  arc A340 (66.675, 7.5692) -> (66.675, 7.6708) centre (66.675, 7.62) ccw
  line L172 (62.865, 7.62) -> (62.23, 6.985)
  arc A341 (60.2891, 5.0441) -> (60.3609, 5.1159) centre (60.325, 5.08) ccw
  arc A342 (59.6541, 6.9491) -> (59.7259, 7.0209) centre (59.69, 6.985) ccw
  arc A343 (64.7341, 7.0209) -> (64.8059, 6.9491) centre (64.77, 6.985) ccw
  arc A344 (57.1141, 6.9491) -> (57.1859, 7.0209) centre (57.15, 6.985) ccw
  line L173 (60.325, 5.08) -> (61.595, 5.08)
  line L174 (59.69, 6.985) -> (59.055, 7.62)
  arc A345 (61.5591, 5.1159) -> (61.6309, 5.0441) centre (61.595, 5.08) ccw
  arc A346 (60.325, 5.1308) -> (60.325, 5.0292) centre (60.325, 5.08) ccw
  arc A347 (57.785, 5.1308) -> (57.785, 5.0292) centre (57.785, 5.08) ccw
  arc A348 (62.9009, 7.5841) -> (62.8291, 7.6559) centre (62.865, 7.62) ccw
  line L175 (66.675, 7.62) -> (65.405, 7.62)
  arc A349 (55.245, 7.6708) -> (55.245, 7.5692) centre (55.245, 7.62) ccw
  line L176 (61.595, 7.62) -> (60.325, 7.62)
  arc A350 (56.515, 7.5692) -> (56.515, 7.6708) centre (56.515, 7.62) ccw
  arc A351 (59.6541, 7.0209) -> (59.7259, 6.9491) centre (59.69, 6.985) ccw
  arc A352 (65.3691, 5.0441) -> (65.4409, 5.1159) centre (65.405, 5.08) ccw
  line L177 (61.595, 5.08) -> (62.23, 5.715)
  arc A353 (55.2091, 5.0441) -> (55.2809, 5.1159) centre (55.245, 5.08) ccw
  arc A354 (53.975, 5.0292) -> (53.975, 5.1308) centre (53.975, 5.08) ccw
  arc A355 (57.1141, 7.0209) -> (57.1859, 6.9491) centre (57.15, 6.985) ccw
  line L178 (64.77, 6.985) -> (65.405, 7.62)
  arc A356 (59.7259, 5.6791) -> (59.6541, 5.7509) centre (59.69, 5.715) ccw
  arc A357 (59.7259, 5.7509) -> (59.6541, 5.6791) centre (59.69, 5.715) ccw
  arc A358 (60.325, 7.6708) -> (60.325, 7.5692) centre (60.325, 7.62) ccw
  arc A359 (57.8209, 7.5841) -> (57.7491, 7.6559) centre (57.785, 7.62) ccw
  arc A360 (69.8141, 6.9491) -> (69.8859, 7.0209) centre (69.85, 6.985) ccw
  line L179 (62.23, 6.985) -> (61.595, 7.62)
  arc A361 (62.1941, 6.9491) -> (62.2659, 7.0209) centre (62.23, 6.985) ccw
  arc A362 (62.1941, 7.0209) -> (62.2659, 6.9491) centre (62.23, 6.985) ccw
  line L180 (57.15, 6.985) -> (57.785, 7.62)
  line L181 (57.785, 5.08) -> (57.15, 5.715)
  line L182 (55.245, 7.62) -> (54.61, 6.985)
  arc A363 (60.3609, 7.5841) -> (60.2891, 7.6559) centre (60.325, 7.62) ccw
  arc A364 (61.6309, 7.6559) -> (61.5591, 7.5841) centre (61.595, 7.62) ccw
  arc A365 (56.515, 5.0292) -> (56.515, 5.1308) centre (56.515, 5.08) ccw
  arc A366 (57.1859, 5.7509) -> (57.1141, 5.6791) centre (57.15, 5.715) ccw
  arc A367 (55.2809, 7.5841) -> (55.2091, 7.6559) centre (55.245, 7.62) ccw
  line L183 (65.405, 5.08) -> (64.77, 5.715)
sketch "Bottom Silkscreen" plane through (0, 0, 0) normal (0, 0, 1) x (1, 0, 0)
  arc A0 (64.6974, 49.0665) -> (64.6974, 49.1553) centre (64.6974, 49.1109) ccw
  arc A1 (63.764, 50.3111) -> (63.8529, 50.3111) centre (63.8085, 50.3111) ccw
  arc A2 (63.8084, 50.3111) -> (63.9418, 49.9999) centre (64.2381, 50.3111) ccw
  arc A3 (63.9756, 50.0287) -> (63.9079, 49.9711) centre (63.9418, 49.9999) ccw
  arc A4 (63.8529, 50.3111) -> (63.764, 50.311) centre (63.8085, 50.311) ccw
  arc A5 (65.4177, 49.4665) -> (65.7733, 49.1109) centre (65.7733, 49.4665) ccw
  arc A6 (64.6974, 50.3555) -> (64.2085, 50.7111) centre (64.2085, 50.1972) ccw
  arc A7 (65.4621, 49.4665) -> (65.3732, 49.4665) centre (65.4177, 49.4665) ccw
  arc A8 (65.7733, 49.1553) -> (65.7733, 49.0665) centre (65.7733, 49.1109) ccw
  line L0 (63.9418, 49.9999) -> (64.6974, 49.1109)
  arc A9 (64.2085, 50.7555) -> (64.2085, 50.6667) centre (64.2085, 50.7111) ccw
  arc A10 (64.6551, 50.3418) -> (64.7397, 50.3692) centre (64.6974, 50.3555) ccw
  arc A11 (64.6636, 49.0821) -> (64.7313, 49.1397) centre (64.6975, 49.1109) ccw
  line L1 (65.7733, 49.1109) -> (65.9511, 49.1109)
  arc A12 (63.8084, 49.1553) -> (63.8084, 49.0665) centre (63.8084, 49.1109) ccw
  arc A13 (65.9511, 49.0665) -> (65.9511, 49.1553) centre (65.9511, 49.1109) ccw
  arc A14 (63.9111, 49.9677) -> (63.9724, 50.0321) centre (63.9418, 49.9999) ccw
  arc A15 (64.2085, 50.7111) -> (63.8084, 50.3111) centre (64.2085, 50.311) ccw
  line L2 (64.6974, 49.1109) -> (63.8084, 49.1109)
  arc A16 (65.4621, 50.7111) -> (65.3732, 50.7111) centre (65.4177, 50.7111) ccw
  arc A17 (28.0289, 5.2134) -> (28.0289, 5.1244) centre (28.0289, 5.1689) ccw
  arc A18 (29.9938, 5.2134) -> (29.9938, 5.1244) centre (29.9938, 5.1689) ccw
  arc A19 (28.9179, 5.1244) -> (28.9179, 5.2134) centre (28.9179, 5.1689) ccw
  line L3 (29.9938, 5.1689) -> (30.1716, 5.1689)
  arc A20 (28.5179, 6.7691) -> (28.429, 6.7691) centre (28.4735, 6.7691) ccw
  arc A21 (29.6382, 5.5245) -> (29.9938, 5.1689) centre (29.9938, 5.5245) ccw
  arc A22 (28.5012, 6.8038) -> (28.4456, 6.7344) centre (28.4734, 6.7691) ccw
  line L4 (28.9179, 5.1689) -> (28.0289, 5.1689)
  line L5 (28.4734, 6.7691) -> (28.4734, 5.1689)
  arc A23 (29.9938, 5.1244) -> (29.9938, 5.2134) centre (29.9938, 5.1689) ccw
  arc A24 (28.429, 5.1689) -> (28.5179, 5.1689) centre (28.4735, 5.1689) ccw
  arc A25 (30.1716, 5.1244) -> (30.1716, 5.2134) centre (30.1716, 5.1689) ccw
  arc A26 (29.5937, 5.5245) -> (29.6826, 5.5245) centre (29.6382, 5.5245) ccw
  arc A27 (29.6826, 5.5245) -> (29.5937, 5.5245) centre (29.6382, 5.5245) ccw
  arc A28 (64.2085, 50.6667) -> (64.2085, 50.7555) centre (64.2085, 50.7111) ccw
  arc A29 (65.3732, 49.4665) -> (65.4621, 49.4665) centre (65.4177, 49.4665) ccw
  arc A30 (28.8901, 6.3788) -> (28.9457, 6.4482) centre (28.9179, 6.4135) ccw
  arc A31 (29.6826, 6.7691) -> (29.5937, 6.7691) centre (29.6382, 6.7691) ccw
  line L6 (65.4177, 50.7111) -> (65.4177, 49.4665)
  arc A32 (65.7733, 49.0665) -> (65.7733, 49.1553) centre (65.7733, 49.1109) ccw
  line L7 (29.6382, 6.7691) -> (29.6382, 5.5245)
  line L8 (28.9179, 6.4135) -> (28.4734, 6.7691)